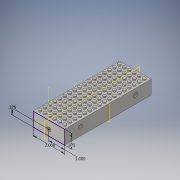
# Autodesk Inventor part: Caufield_Engine_Body_LEGO
Saved by Autodesk Inventor 2016 (Build 200138000, 138)
## iProperties
Created: 2018-01-12
Part Number: Caufield_Engine_Body_LEGO
Material: Generic
Document SubType Name: Modeling
Designer: caufield58738
Density: 1 g/cm^3
Appearance: Default
Author: caufield58738
Autodesk Inventor part; units mm, degrees
ref_plane "YZ Plane" through (0, 0, 0) normal (1, 0, 0) x (0, 1, 0)
ref_plane "XZ Plane" through (0, 0, 0) normal (0, 1, 0) x (-1, 0, 0)
ref_plane "XY Plane" through (0, 0, 0) normal (0, 0, 1) x (1, 0, 0)
sketch "Train Body sketch" plane through (0, 0, 0) normal (0, 0, 1) x (1, 0, 0)
  line L0 (0, 0) -> (50.8, 0)
  line L1 (50.8, 0) -> (50.8, 22.225)
  line L2 (50.8, 22.225) -> (0, 22.225)
  line L3 (0, 22.225) -> (0, 0)
  line L4 (0, 0) -> (50.8, 0)
  line L5 (25.4, 0) -> (25.4, 69.215) construction
  point P0 (25.4, 9.525)
  point P1 (25.4, 9.525)
  dimension "d2" = 50.8
  dimension "d4" = 22.225
  dimension "d5" = 9.525
  dimension "d6" = 25.4
  constraints: 12 end point, 2 horizontal, 2 parallel, 1 midpoint, 1 perpendicular
  measures "d2" distance of L0.start L0.end
  measures "d4" distance of L0.end L1.end
  measures "d5" distance from line of point (25.4, 9.525) L0
  measures "d6" distance from line of L1 point (25.4, 9.525)
extrude "Extrusion4" add sketch "Train Body sketch" against normal blind 139.7
sketch "Sketch6" plane through (50.8, 0, 0) normal (1, 0, 0) x (0, 0, -1)
  line L0 (139.7, 22.225) -> (139.7, 0) projected
  line L1 (0, 0) -> (139.7, 0) projected
  point P0 (25.4, 12.7)
  point P1 (114.3, 12.7)
  dimension "d103" = 114.3
  dimension "d104" = 25.4
  dimension "d105" = 12.7
  constraints: 1 horizontal alignment
  measures "d103" distance from line of L0 point (25.4, 12.7)
  measures "d104" distance from line of L0 point (114.3, 12.7)
  measures "d105" distance from line of L1 point (114.3, 12.7)
ref_plane "Work Plane3" through (25.4, 0, 0) normal (1, 0, 0) x (0, 0, -1)
hole "Hole6" at (50.8, 12.7, -25.4) at (50.8, 12.7, -114.3) direction (-1, 0, 0) diameter 6.35 depth 22.225 tip angle 118
thread "Thread7" size "1/4-20 UNC" class "2B" standard "ANSI Unified Screw Threads" full length
thread "Thread8" size "1/4-20 UNC" class "2B" standard "ANSI Unified Screw Threads" full length
mirror "Mirror2" about plane through (25.4, 0, 0) normal (1, 0, 0) of "Hole6"
thread "Thread9" size "1/4-20 UNC" class "2B" standard "ANSI Unified Screw Threads" full length
thread "Thread10" size "1/4-20 UNC" class "2B" standard "ANSI Unified Screw Threads" full length
hole "Hole7" at (25.4, 9.525, 0) direction (0, 0, -1) diameter 6.35 depth 12.7 tip angle 118
ref_plane "Work Plane4" through (0, 0, -69.85) normal (0, 0, 1) x (1, 0, 0)
mirror "Mirror3" about plane through (0, 0, -69.85) normal (0, 0, 1) of "Hole7"
sketch "Sketch7" plane through (0, 22.225, 0) normal (0, 1, 0) x (1, 0, 0)
  circle A0 centre (5.4, 5.85) radius 2.4
  line L0 (50.8, 0) -> (0, 0) projected
  line L1 (0, 0) -> (0, 139.7) projected
  circle A1 centre (5.4, 13.85) radius 2.4
  circle A2 centre (5.4, 21.85) radius 2.4
  circle A3 centre (5.4, 29.85) radius 2.4
  circle A4 centre (5.4, 37.85) radius 2.4
  circle A5 centre (5.4, 45.85) radius 2.4
  circle A6 centre (5.4, 53.85) radius 2.4
  circle A7 centre (5.4, 61.85) radius 2.4
  circle A8 centre (5.4, 69.85) radius 2.4
  circle A9 centre (5.4, 77.85) radius 2.4
  circle A10 centre (5.4, 85.85) radius 2.4
  circle A11 centre (5.4, 93.85) radius 2.4
  circle A12 centre (5.4, 101.85) radius 2.4
  circle A13 centre (5.4, 109.85) radius 2.4
  circle A14 centre (5.4, 117.85) radius 2.4
  circle A15 centre (5.4, 125.85) radius 2.4
  circle A16 centre (5.4, 133.85) radius 2.4
  circle A17 centre (13.4, 5.85) radius 2.4
  circle A18 centre (13.4, 13.85) radius 2.4
  circle A19 centre (13.4, 21.85) radius 2.4
  circle A20 centre (13.4, 29.85) radius 2.4
  circle A21 centre (13.4, 37.85) radius 2.4
  circle A22 centre (13.4, 45.85) radius 2.4
  circle A23 centre (13.4, 53.85) radius 2.4
  circle A24 centre (13.4, 61.85) radius 2.4
  circle A25 centre (13.4, 69.85) radius 2.4
  circle A26 centre (13.4, 77.85) radius 2.4
  circle A27 centre (13.4, 85.85) radius 2.4
  circle A28 centre (13.4, 93.85) radius 2.4
  circle A29 centre (13.4, 101.85) radius 2.4
  circle A30 centre (13.4, 109.85) radius 2.4
  circle A31 centre (13.4, 117.85) radius 2.4
  circle A32 centre (13.4, 125.85) radius 2.4
  circle A33 centre (13.4, 133.85) radius 2.4
  circle A34 centre (21.4, 5.85) radius 2.4
  circle A35 centre (21.4, 13.85) radius 2.4
  circle A36 centre (21.4, 21.85) radius 2.4
  circle A37 centre (21.4, 29.85) radius 2.4
  circle A38 centre (21.4, 37.85) radius 2.4
  circle A39 centre (21.4, 45.85) radius 2.4
  circle A40 centre (21.4, 53.85) radius 2.4
  circle A41 centre (21.4, 61.85) radius 2.4
  circle A42 centre (21.4, 69.85) radius 2.4
  circle A43 centre (21.4, 77.85) radius 2.4
  circle A44 centre (21.4, 85.85) radius 2.4
  circle A45 centre (21.4, 93.85) radius 2.4
  circle A46 centre (21.4, 101.85) radius 2.4
  circle A47 centre (21.4, 109.85) radius 2.4
  circle A48 centre (21.4, 117.85) radius 2.4
  circle A49 centre (21.4, 125.85) radius 2.4
  circle A50 centre (21.4, 133.85) radius 2.4
  circle A51 centre (29.4, 5.85) radius 2.4
  circle A52 centre (29.4, 13.85) radius 2.4
  circle A53 centre (29.4, 21.85) radius 2.4
  circle A54 centre (29.4, 29.85) radius 2.4
  circle A55 centre (29.4, 37.85) radius 2.4
  circle A56 centre (29.4, 45.85) radius 2.4
  circle A57 centre (29.4, 53.85) radius 2.4
  circle A58 centre (29.4, 61.85) radius 2.4
  circle A59 centre (29.4, 69.85) radius 2.4
  circle A60 centre (29.4, 77.85) radius 2.4
  circle A61 centre (29.4, 85.85) radius 2.4
  circle A62 centre (29.4, 93.85) radius 2.4
  circle A63 centre (29.4, 101.85) radius 2.4
  circle A64 centre (29.4, 109.85) radius 2.4
  circle A65 centre (29.4, 117.85) radius 2.4
  circle A66 centre (29.4, 125.85) radius 2.4
  circle A67 centre (29.4, 133.85) radius 2.4
  circle A68 centre (37.4, 5.85) radius 2.4
  circle A69 centre (37.4, 13.85) radius 2.4
  circle A70 centre (37.4, 21.85) radius 2.4
  circle A71 centre (37.4, 29.85) radius 2.4
  circle A72 centre (37.4, 37.85) radius 2.4
  circle A73 centre (37.4, 45.85) radius 2.4
  circle A74 centre (37.4, 53.85) radius 2.4
  circle A75 centre (37.4, 61.85) radius 2.4
  circle A76 centre (37.4, 69.85) radius 2.4
  circle A77 centre (37.4, 77.85) radius 2.4
  circle A78 centre (37.4, 85.85) radius 2.4
  circle A79 centre (37.4, 93.85) radius 2.4
  circle A80 centre (37.4, 101.85) radius 2.4
  circle A81 centre (37.4, 109.85) radius 2.4
  circle A82 centre (37.4, 117.85) radius 2.4
  circle A83 centre (37.4, 125.85) radius 2.4
  circle A84 centre (37.4, 133.85) radius 2.4
  circle A85 centre (45.4, 5.85) radius 2.4
  circle A86 centre (45.4, 13.85) radius 2.4
  circle A87 centre (45.4, 21.85) radius 2.4
  circle A88 centre (45.4, 29.85) radius 2.4
  circle A89 centre (45.4, 37.85) radius 2.4
  circle A90 centre (45.4, 45.85) radius 2.4
  circle A91 centre (45.4, 53.85) radius 2.4
  circle A92 centre (45.4, 61.85) radius 2.4
  circle A93 centre (45.4, 69.85) radius 2.4
  circle A94 centre (45.4, 77.85) radius 2.4
  circle A95 centre (45.4, 85.85) radius 2.4
  circle A96 centre (45.4, 93.85) radius 2.4
  circle A97 centre (45.4, 101.85) radius 2.4
  circle A98 centre (45.4, 109.85) radius 2.4
  circle A99 centre (45.4, 117.85) radius 2.4
  circle A100 centre (45.4, 125.85) radius 2.4
  circle A101 centre (45.4, 133.85) radius 2.4
  line L2 (0, 139.7) -> (50.8, 139.7) projected
  line L3 (0, 0) -> (50.8, 0) construction
  line L4 (29.4, 0) -> (29.4, 15.8368) construction
  line L5 (25.4, 0) -> (25.4, 16.25) construction
  dimension "d132" = 4.8
  dimension "d133" = 5.85
  dimension "d137" = 8
  dimension "d140" = 8
  dimension "d144" = 4
  constraints: 102 centre point, 4 end point, 2 point on line, 2 vertical, 1 horizontal, 1 midpoint, 1 perpendicular, 202 other
  measures "d132" diameter of A0
  measures "d133" distance from line of L0 A0.centre
  measures "d137" distance of A0.centre A1.centre
  measures "d140" distance of A0.centre A17.centre
  measures "d144" distance between parallel lines of L4 L5
extrude "Extrusion5" add sketch "Sketch7" along normal blind 1.8
body "Solid2"
